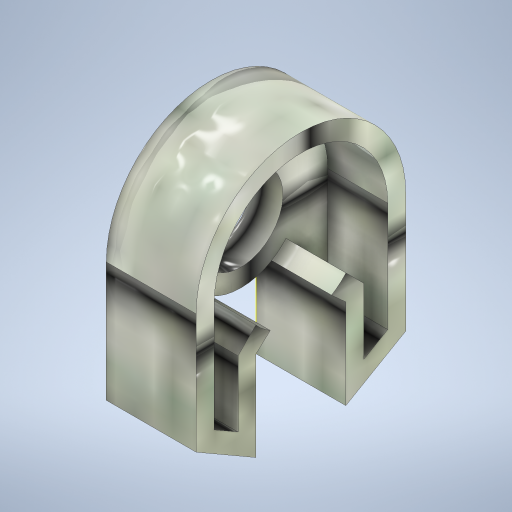
# Autodesk Inventor part: Brazo 3D
Saved by Autodesk Inventor 2023 (Build 270158000, 158)
## iProperties
Created: 2022-10-08
Part Number: Brazo 3D
Material: Generic
Document SubType Name: Modeling
Designer: User
Density: 1 g/cm^3
Appearance: Flat - Gray 1
Author: User
## iProperties of the stored document Brazo_3DPrint.ipt
Created: 2022-10-19
Part Number: Brazo_3DPrint
Material: Generic
Document SubType Name: Modeling
Designer: User
Density: 1 g/cm^3
Appearance: Default
Author: User
Autodesk Inventor part; units mm, degrees
ref_plane "YZ Plane" through (0, 0, 0) normal (1, 0, 0) x (0, 1, 0)
ref_plane "XZ Plane" through (0, 0, 0) normal (0, 1, 0) x (-1, 0, 0)
ref_plane "XY Plane" through (0, 0, 0) normal (0, 0, 1) x (1, 0, 0)
sketch "Sketch1" plane through (0, 0, 0) normal (1, 0, 0) x (0, 1, 0)
  arc A0 (0, -35) -> (0, 35) centre (0, 0) ccw
  circle A1 centre (0, 0) radius 20
  circle A2 centre (0, 0) radius 14
  line L0 (0, 35) -> (-40, 35)
  line L1 (-40, 35) -> (-51.547, 15)
  line L2 (-40, 35) -> (-40, 2.9908) construction
  line L3 (-51.547, 15) -> (-21.547, 15)
  line L4 (-21.547, 15) -> (-17.1937, 10.2166)
  line L5 (0, 0) -> (45.2071, 0) construction
  arc A3 (0, -29) -> (0, 29) centre (0, 0) ccw
  line L6 (0, 29) -> (-36.5359, 29)
  line L7 (-36.5359, 29) -> (-41.1547, 21)
  line L8 (-41.1547, 21) -> (-19.152, 21)
  line L9 (-19.152, 21) -> (-13.1879, 15.0359)
  line L10 (-19.152, 21) -> (-10.7175, 21) construction
  line L11 (0, -35) -> (-40, -35)
  line L12 (-40, -35) -> (-51.547, -15)
  line L13 (-40, -35) -> (-40, -2.9908) construction
  line L14 (-51.547, -15) -> (-21.547, -15)
  line L15 (-21.547, -15) -> (-17.1937, -10.2166)
  line L16 (0, -29) -> (-36.5359, -29)
  line L17 (-36.5359, -29) -> (-41.1547, -21)
  line L18 (-41.1547, -21) -> (-19.152, -21)
  line L19 (-19.152, -21) -> (-13.1879, -15.0359)
  point P0 (0, -29)
  point P1 (-13.1879, -15.0359)
  point P2 (-17.1937, -10.2166)
  dimension "d0" = 70
  dimension "d9" = 15
  dimension "d17" = 6
  dimension "d32" = 40
  dimension "d43" = 20
  dimension "d44" = 30
  dimension "d45" = 30
  dimension "d47" = 6
  dimension "d48" = 45
  dimension "d49" = 132.305
  dimension "d50" = 1.3067
  dimension "d51" = 30.6595
  dimension "d52" = 29
  dimension "d53" = 35
  dimension "d54" = 2.9907
  constraints: 40 end point, 11 symmetric about line, 6 point on circle, 4 centre point, 4 horizontal, 3 coincident, 1 equal length, 1 tangent, 1 vertical, 3 other
  measures "d0" diameter of A0
  measures "d9" radial gap between concentric circles of A0 A1
  measures "d17" radial gap between concentric circles of A1 A2
  measures "d32" distance of L0.start L0.end
  measures "d43" vertical distance of L0.end L1.end
  measures "d44" angle of L2 L1
  measures "d45" distance of L1.end L3.end
  measures "d47" radial gap between concentric circles of A0 A3
  measures "d48" angle of L9 L10
  measures "d49" angle of L5 L15
  measures "d50" distance from line of point (0, 0) L19
  measures "d51" distance from line of L5.end L19
  measures "d52" distance from line of A3.start L5
  measures "d53" distance from line of A0.start L5
  measures "d54" distance from line of L13.end L5
extrude "Extrusion3" add sketch "Sketch1" along normal blind 30 contours L11 L12 L14 L15 A1 L19 L18 L17 L16 A3 L6 L7 L8 L9 L4 L3 L1 L0 A0
extrude "Extrusion4" add sketch "Sketch1" along normal blind 10 contours A1 | A1 L9 L8 L7 L6 A3 L16 L17 L18 L19
sketch "Sketch2" plane through (0, 0, 0) normal (-1, 0, 0) x (0, 0, 1)
  line L0 (-15, -21.547) -> (-15, -51.547) projected
  line L1 (-10.2166, -17.1937) -> (-15, -21.547) projected
  line L2 (-15, -21.547) -> (-10.2166, -17.1937)
  arc A0 (-10.2166, -17.1937) -> (10.2166, -17.1937) centre (0, 0) ccw projected
  arc A1 (-10.2166, -17.1937) -> (10.2166, -17.1937) centre (0, 0) ccw
  line L3 (15, -51.547) -> (15, -21.547) projected
  line L4 (15, -21.547) -> (10.2166, -17.1937) projected
  line L5 (15, -21.547) -> (10.2166, -17.1937)
  constraints: 4 end point, 2 collinear, 2 point on circle, 1 centre point
body "Solid2"
